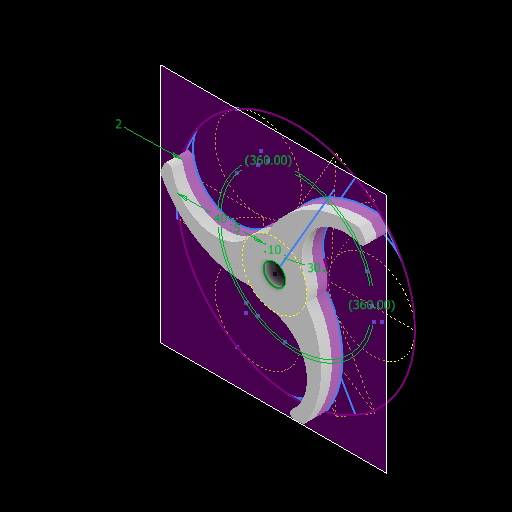
# Autodesk Inventor part: Combine mk5
Saved by Autodesk Inventor 2025 (Build 290162000, 162)
## iProperties
Created: 2024-09-10
Part Number: Combine mk5
Material: Generic
Document SubType Name: Modeling
Designer: Trevor
Density: 1 g/cm^3
Appearance: Default
Author: Trevor
Autodesk Inventor part; units mm, degrees
ref_plane "YZ Plane" through (0, 0, 0) normal (1, 0, 0) x (0, 1, 0)
ref_plane "XZ Plane" through (0, 0, 0) normal (0, 1, 0) x (-1, 0, 0)
ref_plane "XY Plane" through (0, 0, 0) normal (0, 0, 1) x (1, 0, 0)
sketch "Sketch1" plane through (0, 0, 0) normal (0, 0, 1) x (1, 0, 0)
  circle A0 centre (0, 0) radius 15
  circle A1 centre (0, 0) radius 55
  line L0 (15, 0) -> (55, 0) construction
  circle A2 centre (35, 0) radius 20 construction
  circle A3 centre (-17.5, 30.3109) radius 20 construction
  circle A4 centre (-17.5, -30.3109) radius 20 construction
  line L1 (0, 0) -> (-10.834, 10.3742)
  line L2 (0, 0) -> (27.5, -47.6314)
  line L3 (0, 0) -> (-55, 0) construction
  line L4 (0, 0) -> (27.5, 47.6314)
  line L5 (17.5, 30.3109) -> (27.5, 47.6314) construction
  line L6 (-1.4324, 18.1475) -> (18.5676, 52.7885) construction
  line L7 (18.5676, 52.7885) -> (36.4324, 42.4743) construction
  line L8 (36.4324, 42.4743) -> (16.4324, 7.8333) construction
  line L9 (16.4324, 7.8333) -> (-1.4324, 18.1475) construction
  line L10 (-1.4324, 18.1475) -> (36.4324, 42.4743) construction
  line L11 (18.5676, 52.7885) -> (16.4324, 7.8333) construction
  line L12 (-1.4891, -18.1802) -> (18.5109, -52.8212) construction
  line L13 (18.5109, -52.8212) -> (36.4891, -42.4416) construction
  line L14 (36.4891, -42.4416) -> (16.4891, -7.8006) construction
  line L15 (16.4891, -7.8006) -> (-1.4891, -18.1802) construction
  line L16 (-1.4891, -18.1802) -> (36.4891, -42.4416) construction
  line L17 (18.5109, -52.8212) -> (16.4891, -7.8006) construction
  line L18 (-55.0081, 10.3109) -> (-15, 10.3109) construction
  line L19 (-15, 10.3109) -> (-15, -10.3109) construction
  line L20 (-15, -10.3109) -> (-55.0081, -10.3109) construction
  line L21 (-55.0081, -10.3109) -> (-55.0081, 10.3109)
  line L22 (-55.0081, 10.3109) -> (-15, -10.3109) construction
  line L23 (-15, 10.3109) -> (-55.0081, -10.3109) construction
  line L24 (-39.1178, -2.5) -> (-30.8902, -2.5) construction
  line L25 (-30.8902, -2.5) -> (-30.8902, 2.5) construction
  line L26 (-30.8902, 2.5) -> (-39.1178, 2.5) construction
  line L27 (-39.1178, 2.5) -> (-39.1178, -2.5) construction
  line L28 (-39.1178, -2.5) -> (-30.8902, 2.5) construction
  line L29 (-30.8902, -2.5) -> (-39.1178, 2.5) construction
  line L30 (-55.0081, 10.3109) -> (-55.0081, -10.3109) construction
  line L31 (-55.0081, 10.3109) -> (-55.0081, -10.3109) construction
  circle A5 centre (0, 0) radius 5
  arc A6 (-47.6318, 23.7685) -> (-10.834, 10.3742) centre (-27.4698, 21.9149) ccw
  line L32 (-15, -10.3109) -> (-10.8943, -10.3109)
  line L33 (-46.714, 28.5112) -> (-52.5923, 15.6119)
  arc A7 (-52.5567, 13.8792) -> (-17.5, -10.3109) centre (-12.7886, 34.0144) ccw
  arc A8 (-17.5, -10.3109) -> (-15, -10.3109) centre (-16.25, 36.3845) ccw
  arc A9 (-52.5923, 15.6119) -> (-52.5567, 13.8792) centre (-50.7724, 14.7826) ccw
  line L34 (-46.714, 28.5112) -> (-45.8939, 30.3109)
  arc A10 (-45.8939, 30.3109) -> (-47.6318, 23.7685) centre (-27.4698, 21.9149) ccw
  arc A11 (14.2587, -52.455) -> (17.6795, -10) centre (-23.063, -28.0825) ccw
  arc A12 (12.7758, -53.3523) -> (14.2587, -52.455) centre (12.5841, -51.3615) ccw
  line L35 (-1.3344, -54.7111) -> (12.7758, -53.3523)
  arc A13 (3.2318, -53.1346) -> (-3.5673, -14.5696) centre (-5.2439, -34.747) ccw
  arc A14 (-3.3031, -54.9007) -> (3.2318, -53.1346) centre (-5.2439, -34.747) ccw
  line L36 (-1.3344, -54.7111) -> (-3.3031, -54.9007)
  line L37 (16.4295, -7.8349) -> (14.3766, -4.2793)
  arc A15 (17.6795, -10) -> (16.4295, -7.8349) centre (-23.3849, -32.2652) ccw
  circle A16 centre (0, 0) radius 15
  arc A17 (38.2981, 38.5759) -> (-0.1795, 20.3109) centre (35.8517, -5.9319) ccw
  arc A18 (39.8165, 37.7403) -> (38.2981, 38.5759) centre (38.1883, 36.5789) ccw
  line L38 (48.0484, 26.2) -> (39.8165, 37.7403)
  arc A19 (44.4, 29.3661) -> (14.4013, 4.1954) centre (32.7138, 12.8321) ccw
  arc A20 (49.1969, 24.5898) -> (44.4, 29.3661) centre (32.7138, 12.8321) ccw
  line L39 (48.0484, 26.2) -> (49.1969, 24.5898)
  line L40 (-1.4295, 18.1458) -> (-3.4823, 14.5902)
  arc A21 (-0.1795, 20.3109) -> (-1.4295, 18.1458) centre (39.6349, -4.1193) ccw
  circle A22 centre (0, 0) radius 15
  point P0 (-27.5, 47.6314)
  point P1 (-27.5, -47.6314)
  point P2 (17.5, -30.3109)
  point P3 (-35.004, 0)
  point P4 (-52.9855, 14.7493)
  point P5 (-52.9855, 14.7493)
  point P6 (7.5, -12.9904)
  point P7 (-12.5218, 8.2586)
  point P8 (-7.5, 12.9904)
  point P9 (-7.5, -12.9904)
  point P10 (-0.8912, -14.9735)
  point P11 (13.413, 6.7149)
  dimension "d0" = 30
  dimension "d1" = 40
  dimension "d4" = 360
  dimension "d6" = 5
  dimension "d11" = 10
  dimension "d24" = 2
  dimension "d31" = 360
  constraints: 82 end point, 49 point on circle, 20 centre point, 10 point on line, 9 midpoint, 9 parallel, 4 perpendicular, 3 coincident, 3 horizontal, 3 tangent, 1 concentric, 1 horizontal alignment, 95 other
  measures "d0" diameter of A0
  measures "d1" radial gap between concentric circles of A0 A1
  measures "d6" distance of L25.end L24.end
  measures "d11" radial gap between concentric circles of A0 A5
  measures "d24" radius of A9
extrude "Extrusion1" add sketch "Sketch1" along normal blind 10 contours A0 L2 A5 L4 A19 | A19 A0 | L37 A15 A11 L2 A0 | A0 L4 A17 A18 L38 L39 A20 A19 | L2 A11 A12 L35 L36 A14 A13 A0 | A0 A13 A6 L1 A5 L2 | L4 A5 L1 A0 | A0 L40 A21 A17 L4 | A0 A13 | A6 A0 | L32 A8 A7 A9 L33 L34 A10 A6 A0
fillet "Fillet1" radius 2 3 edges at (-45.8939, 30.3109, 5) (49.1969, 24.5898, 5) (-3.3031, -54.9007, 5)
sketch "Sketch2" plane through (0, 0, 10) normal (0, 0, 1) x (1, 0, 0)
  line L0 (17.5, 30.3109) -> (27.5, 47.6314) construction
  line L1 (27.5, 47.6314) -> (2.5, 4.3301)
  circle A0 centre (0, 0) radius 5 projected
  circle A1 centre (0, 0) radius 15 construction
  circle A2 centre (0, 0) radius 5 construction
  constraints: 2 coincident, 2 end point, 1 centre point, 5 other
ref_plane "Work Plane3" through (0, 0, 5) normal (0, 0, -1) x (-1, 0, 0)
body "Solid1"
